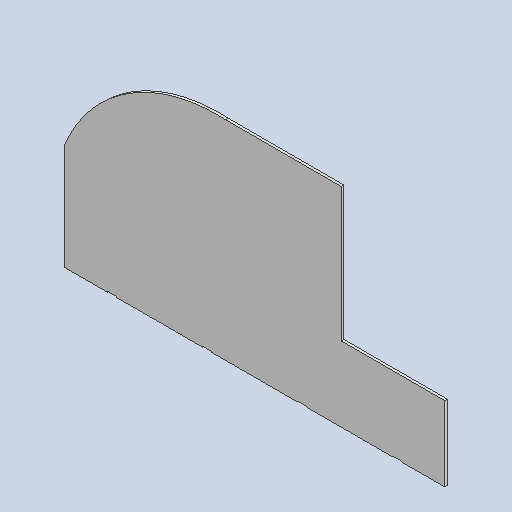
# Autodesk Inventor part: 사이드 카울
Saved by Autodesk Inventor 2025.2 (Build 292293000, 293)
## iProperties
Created: 2025-07-11
Part Number: 사이드 카울
Material: 일반
Document SubType Name: Modeling
Designer: jbhma
Density: 1 g/cm^3
Appearance: 기본값
Author: jbhma
Autodesk Inventor part; units mm, degrees
ref_plane "YZ Plane" through (0, 0, 0) normal (1, 0, 0) x (0, 1, 0)
ref_plane "XZ Plane" through (0, 0, 0) normal (0, 1, 0) x (-1, 0, 0)
ref_plane "XY Plane" through (0, 0, 0) normal (0, 0, 1) x (1, 0, 0)
sketch "스케치1" plane through (0, 0, 0) normal (0, 0, 1) x (1, 0, 0)
  line L0 (552.9734, 795) -> (1055, 795)
  line L1 (1450, 285) -> (1450, 0)
  line L2 (1450, 0) -> (0, 0)
  line L3 (0, 0) -> (0, 405)
  line L4 (0, 0) -> (0, 405) construction
  arc A0 (614, 795) -> (0, 405) centre (583.4867, 164.7107) ccw
  line L5 (1450, 285) -> (1055, 285)
  line L6 (1055, 0) -> (1450, 0)
  line L7 (1450, 0) -> (1450, 285)
  line L8 (1055, 285) -> (1055, 795)
  dimension "d0" = 1450
  dimension "d2" = 405
  dimension "d3" = 631.0275
  dimension "d4" = 836
  dimension "d7" = 285
  dimension "d9" = 395
  dimension "d10" = 510
  dimension "d11" = 395
  constraints: 18 end point, 4 parallel, 3 point on circle, 2 horizontal, 2 perpendicular, 2 point on line, 1 centre point, 1 coincident
  measures "d0" distance of L1.end L2.end
  measures "d2" distance of L3.end L2.end
  measures "d3" radius of A0
  measures "d4" distance from line of A0.start L1
  measures "d7" distance between parallel lines of L2 L5
  measures "d9" distance between parallel lines of L8 L1
  measures "d10" distance between parallel lines of L5 L0
  measures "d11" distance from line of L6.start L1
extrude "돌출1" add sketch "스케치1" along normal blind 10
sketch "스케치3" plane through (0, 0, 10) normal (0, 0, 1) x (1, 0, 0)
  line L0 (0, 0) -> (1450, 0) projected
  line L1 (1450, 0) -> (1450, 285) projected
  line L2 (1450, 285) -> (1055, 285) projected
  line L3 (1055, 285) -> (1055, 795) projected
  line L4 (1055, 795) -> (614, 795) projected
  arc A0 (614, 795) -> (0, 405) centre (583.4867, 164.7107) ccw projected
  line L5 (0, 405) -> (0, 0) projected
  line L6 (725, 0) -> (725, 795) construction
  line L7 (362.5, 0) -> (362.5, 755.778) construction
  line L8 (1087.5, 0) -> (1087.5, 285) construction
  line L9 (181.25, 0) -> (181.25, 650.9219) construction
  line L10 (543.75, 0) -> (543.75, 794.4858) construction
  line L11 (906.25, 0) -> (906.25, 795) construction
  line L12 (1268.75, 0) -> (1268.75, 285) construction
  line L13 (163.75, 0) -> (198.75, 0)
  line L14 (198.75, 0) -> (198.75, 3)
  line L15 (198.75, 3) -> (163.75, 3)
  line L16 (163.75, 3) -> (163.75, 0)
  line L17 (526.25, 0) -> (561.25, 0)
  line L18 (561.25, 0) -> (561.25, 3)
  line L19 (561.25, 3) -> (526.25, 3)
  line L20 (526.25, 3) -> (526.25, 0)
  line L21 (888.75, 0) -> (923.75, 0)
  line L22 (923.75, 0) -> (923.75, 3)
  line L23 (923.75, 3) -> (888.75, 3)
  line L24 (888.75, 3) -> (888.75, 0)
  line L25 (1251.25, 0) -> (1286.25, 0)
  line L26 (1286.25, 0) -> (1286.25, 3)
  line L27 (1286.25, 3) -> (1251.25, 3)
  line L28 (1251.25, 3) -> (1251.25, 0)
  point P0 (181.25, 3)
  point P1 (543.75, 3)
  point P2 (906.25, 3)
  point P3 (1268.75, 3)
  dimension "d14" = 725
  dimension "d15" = 362.5
  dimension "d16" = 362.5
  dimension "d17" = 181.25
  dimension "d18" = 181.25
  dimension "d19" = 181.25
  dimension "d20" = 181.25
  dimension "d21" = 35
  dimension "d22" = 3
  dimension "d23" = 35
  dimension "d24" = 3
  dimension "d25" = 35
  dimension "d26" = 3
  dimension "d27" = 35
  dimension "d28" = 3
  constraints: 46 end point, 10 parallel, 8 perpendicular, 8 point on line, 4 horizontal, 4 midpoint, 3 point on circle, 1 vertical, 12 other
  measures "d14" distance between parallel lines of L6 L5
  measures "d15" distance between parallel lines of L7 L5
  measures "d16" distance between parallel lines of L8 L1
  measures "d17" distance between parallel lines of L9 L5
  measures "d18" distance between parallel lines of L10 L7
  measures "d19" distance between parallel lines of L11 L6
  measures "d20" distance between parallel lines of L12 L1
  measures "d21" distance of L15.end L14.end
  measures "d22" distance of L14.end L13.end
  measures "d23" distance of L19.end L18.end
  measures "d24" distance of L18.end L17.end
  measures "d25" distance of L23.end L22.end
  measures "d26" distance of L22.end L21.end
  measures "d27" distance of L27.end L26.end
  measures "d28" distance of L26.end L25.end
extrude "돌출2" cut sketch "스케치3" against normal blind 10 contours L16 L15 L14 L0 | L20 L19 L18 L0 | L24 L23 L22 L0 | L28 L27 L26 L0
